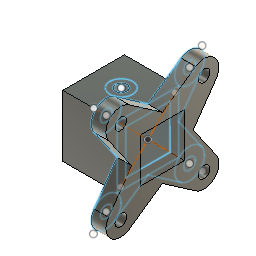
Motor-mainrod fitting v5 (Autodesk Fusion 360 design; units mm, degrees)
Autodesk Fusion 360 part; units mm, degrees
sketch "Sketch2" plane through (5, 0, 0) normal (1, 0, 0) x (0, 1, 0)
  line L0 (16.9637, 18.2844) -> (-13.0292, -11.7227) construction
  line L1 (-12.9363, 18.2856) -> (17.0619, -11.7162) construction
  circle A0 centre (13.5169, 14.8306) radius 1.6
  circle A1 centre (-9.4831, 14.8306) radius 1.6
  circle A2 centre (-9.4831, -8.1694) radius 1.6
  circle A3 centre (13.5169, -8.1694) radius 1.6
  circle A4 centre (-9.4831, 14.8306) radius 4.1
  circle A5 centre (13.5169, 14.8306) radius 4.1
  circle A6 centre (-9.4831, -8.1694) radius 4.1
  line L2 (9.4619, 10.7862) -> (-5.5274, -4.2245) construction
  line L3 (-7.1431, 18.1972) -> (2.0169, 11.8306)
  line L4 (2.0169, 11.8306) -> (11.1769, 18.1972)
  line L5 (-12.8477, 12.4876) -> (-6.471, 3.3306)
  line L6 (-6.471, 3.3306) -> (-12.8477, -5.8265)
  line L7 (-7.1431, -11.5361) -> (2.0169, -5.1694)
  line L8 (10.5048, 3.3306) -> (16.8815, 12.4876)
  circle A7 centre (13.5169, -8.1694) radius 4.1
  line L9 (10.5048, 3.3306) -> (16.8815, -5.8265)
  line L10 (2.0169, -5.1694) -> (11.1769, -11.5361)
  line L11 (-4.0831, -2.7694) -> (8.1169, -2.7694)
  line L12 (8.1169, -2.7694) -> (8.1169, 9.4306)
  line L13 (8.1169, 9.4306) -> (-4.0831, 9.4306)
  line L14 (-4.0831, 9.4306) -> (-4.0831, -2.7694)
  line L15 (-4.0831, -2.7694) -> (8.1169, 9.4306) construction
  line L16 (8.1169, -2.7694) -> (-4.0831, 9.4306) construction
  line L17 (10.5048, 11.8306) -> (-6.471, 11.8306)
  line L18 (-6.471, 11.8306) -> (-6.471, -5.1694)
  line L19 (-6.471, -5.1694) -> (10.5048, -5.1694)
  line L20 (10.5048, -5.1694) -> (10.5048, 11.8306)
  line L21 (10.5048, 11.8306) -> (-6.471, -5.1694) construction
  line L22 (-6.471, 11.8306) -> (10.5048, -5.1694) construction
  point P0 (2.0169, 3.3306)
  point P1 (2.0169, 3.3306)
  point P2 (2.0169, 3.3306)
  point P3 (2.0169, 3.3306)
  point P4 (2.0169, 3.3306)
  dimension "d11" = 3.2
  dimension "d12" = 11.5
  dimension "d13" = 3.2
  dimension "d14" = 3.2
  dimension "d15" = 3.2
  dimension "d18" = 11.5
  dimension "d19" = 23
  dimension "d20" = 8.2
  dimension "d21" = 8.2
  dimension "d22" = 8.2
  dimension "d23" = 8.2
  dimension "d33" = 12.2
  dimension "d34" = 17
  dimension "d35" = 23
  constraint coincident L0 P4
  constraint coincident L1 P4
  constraint coincident P4 P3
  constraint horizontal A0.centre A1.centre
  constraint vertical A1.centre A2.centre
  constraint horizontal A2.centre A3.centre
  constraint vertical A0.centre A3.centre
  constraint concentric A1 A4
  constraint concentric A0 A5
  constraint concentric A2 A6
  constraint coincident L2 P4
  constraint coincident A4 L3.start
  constraint tangent A4 L3
  constraint coincident A5 L4.end
  constraint tangent A5 L4
  constraint coincident A4 L5.start
  constraint coincident A6 L6.end
  constraint tangent A6 L6
  constraint tangent A4 L5
  constraint coincident A6 L7.start
  constraint tangent A6 L7
  constraint coincident A5 L8.end
  constraint tangent A5 L8
  constraint concentric A3 A7
  constraint coincident A7 L9.end
  constraint tangent A7 L9
  constraint coincident A7 L10.end
  constraint tangent A7 L10
  constraint horizontal L11
  constraint perpendicular L11 L12
  constraint coincident L15 P4
  constraint coincident L16 P4
  constraint equal L13 L14
  constraint equal L11 L12
  constraint horizontal L17
  constraint perpendicular L17 L18
  constraint parallel L17 L19
  constraint parallel L18 L20
  constraint coincident L21 P4
  constraint coincident L22 P4
  constraint coincident L2 L17.start
  constraint midpoint L7.end L19
  constraint midpoint L8.start L20
  constraint midpoint L3.end L17
  constraint midpoint L5.end L18
  measures "d11" diameter of A0
  measures "d12" horizontal distance of P4 A0.centre
  measures "d13" diameter of A1
  measures "d14" diameter of A2
  measures "d15" diameter of A3
  measures "d18" vertical distance of P4 A0.centre
  measures "d19" vertical distance of A0.centre A3.centre
  measures "d20" diameter of A4
  measures "d21" diameter of A5
  measures "d22" diameter of A6
  measures "d23" diameter of A7
  measures "d33" distance of L11 L13
  measures "d34" distance of L17.end L18.end
  measures "d35" distance of A1.centre A0.centre
extrude "Extrude14" add sketch "Sketch2" along normal blind 5
extrude "Extrude16" add sketch "Sketch2" against normal blind 15 contours L17 L18 L19 L20
sketch "Sketch5" plane through (0, 0, 11.8306) normal (0, 0, 1) x (-1, 0, 0)
  line L0 (-5, -2.0169) -> (-5, -10.5048)
  line L1 (-5, -10.5048) -> (10, -10.5048)
  line L2 (10, -10.5048) -> (10, 6.471)
  line L3 (10, 6.471) -> (-5, 6.471)
  line L4 (-5, 6.471) -> (-5, -2.0169)
  circle A0 centre (2.5, -2.1573) radius 1.6
  circle A1 centre (2.5, -2.1573) radius 3.1
  dimension "d61" = 3.2
  dimension "d64" = 6.2
  constraint concentric A0 A1
  measures "d61" diameter of A0
  measures "d64" diameter of A1
extrude "Extrude17" cut sketch "Sketch5" against normal blind 5 contours A0
move_face "MoveFace1" by (-1, 0, 0) 1 faces at (10, -3.3164, 12.0306)
extrude "Extrude18" [suppressed]
extrude "Extrude15" [suppressed]
extrude "Extrude3" [suppressed]
equation "d11 = motorScrewHole"
equation "d12 = boltDistance / 2"
equation "d13 = motorScrewHole"
equation "d14 = motorScrewHole"
equation "d15 = motorScrewHole"
equation "motorScrewHole = 3.2 mm" comment "poo"
equation "d18 = boltDistance / 2"
equation "d19 = boltDistance"
equation "d20 = motorScrewHole + 5 mm"
equation "d21 = motorScrewHole + 5 mm"
equation "d22 = motorScrewHole + 5 mm"
equation "d23 = motorScrewHole + 5 mm"
equation "d35 = boltDistance"
equation "boltDistance = 23 mm"
